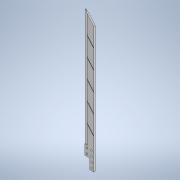
# Autodesk Inventor part: blade D 3.25
Saved by Autodesk Inventor 2021 (Build 250183000, 183)
## iProperties
Created: 2021-04-14
Part Number: blade D 3.25
Material: Generic
Document SubType Name: Modeling
Designer: newic
Density: 1 g/cm^3
Appearance: Default
Author: newic
Autodesk Inventor part; units mm, degrees
ref_plane "YZ Plane" through (0, 0, 0) normal (1, 0, 0) x (0, 1, 0)
ref_plane "XZ Plane" through (0, 0, 0) normal (0, 1, 0) x (-1, 0, 0)
ref_plane "XY Plane" through (0, 0, 0) normal (0, 0, 1) x (1, 0, 0)
sketch "Sketch1" plane through (0, 0, 0) normal (0, 0, 1) x (1, 0, 0)
  line L0 (0, 0) -> (82.55, 0)
  line L1 (82.55, 0) -> (82.55, 968.4207)
  line L2 (82.55, 968.4207) -> (82.55, 804.8513)
  line L3 (82.55, 804.8513) -> (82.55, 621.9713)
  line L4 (82.55, 621.9713) -> (82.55, 439.0913)
  line L5 (82.55, 439.0913) -> (82.55, 256.2113)
  line L6 (82.55, 256.2113) -> (82.55, 73.3313)
  line L7 (0, 1066.8) -> (0, 0)
  line L8 (0, 1066.8) -> (82.55, 968.4207)
  line L9 (-23.6845, 1095.0261) -> (784.1067, 132.338)
  line L10 (-109.2976, 1023.1881) -> (698.4936, 60.5001)
  line L11 (-194.9107, 951.3502) -> (612.8804, -11.3378)
  line L12 (-280.5239, 879.5122) -> (527.2673, -83.1758)
  line L13 (-366.137, 807.6743) -> (441.6542, -155.0137)
  line L14 (-451.7501, 735.8363) -> (356.041, -226.8517)
  dimension "d26" = 1066.8
  dimension "d27" = 82.55
  dimension "d28" = 40
  dimension "d34" = 111.76
  dimension "d35" = 111.76
  dimension "d36" = 111.76
  dimension "d37" = 111.76
  dimension "d38" = 111.76
  constraints: 30 end point, 6 parallel, 6 point on line, 1 horizontal, 1 perpendicular
  measures "d26" distance of L7.start L0.start
  measures "d27" distance of L0.start L0.end
  measures "d28" angle of L8 L1
  measures "d34" distance between parallel lines of L9 L10
  measures "d35" distance between parallel lines of L10 L11
  measures "d36" distance between parallel lines of L11 L12
  measures "d37" distance between parallel lines of L12 L13
  measures "d38" distance between parallel lines of L13 L14
extrude "Extrusion1" add sketch "Sketch1" along normal blind 12.7
sketch "Sketch2" plane through (0, 0, 12.7) normal (0, 0, 1) x (1, 0, 0)
  line L0 (0, 0) -> (82.55, 0)
  line L1 (82.55, 0) -> (82.55, 968.4207)
  line L2 (82.55, 968.4207) -> (82.55, 804.8513)
  line L3 (82.55, 804.8513) -> (82.55, 621.9713)
  line L4 (82.55, 621.9713) -> (82.55, 439.0913)
  line L5 (82.55, 439.0913) -> (82.55, 256.2113)
  line L6 (82.55, 256.2113) -> (82.55, 73.3313)
  line L7 (0, 1066.8) -> (0, 0)
  line L8 (0, 1066.8) -> (82.55, 968.4207)
  line L9 (-23.6845, 1095.0261) -> (784.1067, 132.338)
  line L10 (-109.2976, 1023.1881) -> (698.4936, 60.5001)
  line L11 (-194.9107, 951.3502) -> (612.8804, -11.3378)
  line L12 (-280.5239, 879.5122) -> (527.2673, -83.1758)
  line L13 (-366.137, 807.6743) -> (441.6542, -155.0137)
  line L14 (-451.7501, 735.8363) -> (356.041, -226.8517)
  line L15 (-453.2094, 734.6118) -> (354.5817, -228.0762)
  line L16 (-450.2908, 737.0609) -> (357.5004, -225.6272)
  line L17 (-367.5963, 806.4498) -> (440.1949, -156.2382)
  line L18 (-364.6777, 808.8988) -> (443.1135, -153.7892)
  line L19 (-281.9832, 878.2877) -> (525.808, -84.4003)
  line L20 (-279.0645, 880.7367) -> (528.7266, -81.9513)
  line L21 (-196.37, 950.1257) -> (611.4211, -12.5624)
  line L22 (-193.4514, 952.5747) -> (614.3397, -10.1133)
  line L23 (-110.7569, 1021.9636) -> (697.0342, 59.2756)
  line L24 (-107.8383, 1024.4126) -> (699.9529, 61.7246)
  point P0 (0, 889.9687)
  point P1 (82.55, 791.5894)
  point P2 (82.55, 797.5167)
  point P3 (0, 895.896)
  point P4 (0, 716.101)
  point P5 (82.55, 617.7217)
  point P6 (82.55, 623.649)
  point P7 (0, 722.0283)
  point P8 (0, 542.2333)
  point P9 (82.55, 443.854)
  point P10 (82.55, 449.7813)
  point P11 (0, 548.1606)
  point P12 (0, 368.3656)
  point P13 (82.55, 269.9863)
  point P14 (82.55, 275.9136)
  point P15 (0, 374.2929)
  point P16 (0, 194.4979)
  point P17 (82.55, 96.1186)
  point P18 (82.55, 102.0459)
  point P19 (0, 200.4252)
  dimension "d41" = 1066.8
  dimension "d42" = 82.55
  dimension "d43" = 40
  dimension "d44" = 111.76
  dimension "d45" = 111.76
  dimension "d46" = 111.76
  dimension "d47" = 111.76
  dimension "d48" = 111.76
  dimension "d49" = 1.905
  dimension "d50" = 1.905
  dimension "d51" = 1.905
  dimension "d52" = 1.905
  dimension "d53" = 1.905
  dimension "d54" = 1.905
  dimension "d55" = 1.905
  dimension "d56" = 1.905
  dimension "d57" = 1.905
  dimension "d58" = 1.905
  constraints: 50 end point, 16 parallel, 6 point on line, 1 horizontal, 1 perpendicular
  measures "d41" distance of L7.start L0.start
  measures "d42" distance of L0.start L0.end
  measures "d43" angle of L8 L1
  measures "d44" distance between parallel lines of L9 L10
  measures "d45" distance between parallel lines of L10 L11
  measures "d46" distance between parallel lines of L11 L12
  measures "d47" distance between parallel lines of L12 L13
  measures "d48" distance between parallel lines of L13 L14
  measures "d49" distance between parallel lines of L14 L15
  measures "d50" distance between parallel lines of L14 L16
  measures "d51" distance between parallel lines of L13 L17
  measures "d52" distance between parallel lines of L13 L18
  measures "d53" distance between parallel lines of L12 L19
  measures "d54" distance between parallel lines of L12 L20
  measures "d55" distance between parallel lines of L11 L21
  measures "d56" distance between parallel lines of L11 L22
  measures "d57" distance between parallel lines of L10 L23
  measures "d58" distance between parallel lines of L10 L24
extrude "Extrusion2" cut sketch "Sketch2" against normal blind 12.7 contours L7 L14 L1 L15 | L7 L16 L1 L14 | L7 L13 L1 L17 | L7 L18 L1 L13 | L7 L12 L1 L19 | L7 L20 L1 L12 | L7 L11 L1 L21 | L7 L22 L1 L11 | L7 L10 L1 L23 | L7 L24 L1 L10
sketch "Sketch3" plane through (0, 0, 12.7) normal (0, 0, 1) x (1, 0, 0)
  line L0 (0, 0) -> (82.55, 0)
  line L1 (82.55, 0) -> (82.55, 968.4207)
  line L2 (82.55, 968.4207) -> (82.55, 804.8513)
  line L3 (82.55, 804.8513) -> (82.55, 621.9713)
  line L4 (82.55, 621.9713) -> (82.55, 439.0913)
  line L5 (82.55, 439.0913) -> (82.55, 256.2113)
  line L6 (82.55, 256.2113) -> (82.55, 73.3313)
  line L7 (0, 1066.8) -> (0, 0)
  line L8 (0, 1066.8) -> (82.55, 968.4207)
  line L9 (-23.6845, 1095.0261) -> (784.1067, 132.338)
  line L10 (-109.2976, 1023.1881) -> (698.4936, 60.5001)
  line L11 (-194.9107, 951.3502) -> (612.8804, -11.3378)
  line L12 (-280.5239, 879.5122) -> (527.2673, -83.1758)
  line L13 (-366.137, 807.6743) -> (441.6542, -155.0137)
  line L14 (-451.7501, 735.8363) -> (356.041, -226.8517)
  line L15 (-453.2094, 734.6118) -> (354.5817, -228.0762)
  line L16 (-450.2908, 737.0609) -> (357.5004, -225.6272)
  line L17 (-367.5963, 806.4498) -> (440.1949, -156.2382)
  line L18 (-364.6777, 808.8988) -> (443.1135, -153.7892)
  line L19 (-281.9832, 878.2877) -> (525.808, -84.4003)
  line L20 (-279.0645, 880.7367) -> (528.7266, -81.9513)
  line L21 (-196.37, 950.1257) -> (611.4211, -12.5624)
  line L22 (-193.4514, 952.5747) -> (614.3397, -10.1133)
  line L23 (-110.7569, 1021.9636) -> (697.0342, 59.2756)
  line L24 (-107.8383, 1024.4126) -> (699.9529, 61.7246)
  point P0 (0, 889.9687)
  point P1 (82.55, 791.5894)
  point P2 (82.55, 797.5167)
  point P3 (0, 895.896)
  point P4 (0, 716.101)
  point P5 (82.55, 617.7217)
  point P6 (82.55, 623.649)
  point P7 (0, 722.0283)
  point P8 (0, 542.2333)
  point P9 (82.55, 443.854)
  point P10 (82.55, 449.7813)
  point P11 (0, 548.1606)
  point P12 (0, 368.3656)
  point P13 (82.55, 269.9863)
  point P14 (82.55, 275.9136)
  point P15 (0, 374.2929)
  point P16 (0, 194.4979)
  point P17 (82.55, 96.1186)
  point P18 (82.55, 102.0459)
  point P19 (0, 200.4252)
  point P20 (0, 889.9687)
  point P21 (82.55, 791.5894)
  point P22 (82.55, 797.5167)
  point P23 (0, 895.896)
  point P24 (0, 716.101)
  point P25 (82.55, 617.7217)
  point P26 (82.55, 623.649)
  point P27 (0, 722.0283)
  point P28 (0, 542.2333)
  point P29 (82.55, 443.854)
  point P30 (82.55, 449.7813)
  point P31 (0, 548.1606)
  point P32 (0, 368.3656)
  point P33 (82.55, 269.9863)
  point P34 (82.55, 275.9136)
  point P35 (0, 374.2929)
  point P36 (0, 194.4979)
  point P37 (82.55, 96.1186)
  point P38 (82.55, 102.0459)
  point P39 (0, 200.4252)
  dimension "d114" = 15.875
  dimension "d61" = 1066.8
  dimension "d62" = 82.55
  dimension "d63" = 40
  dimension "d64" = 111.76
  dimension "d65" = 111.76
  dimension "d66" = 111.76
  dimension "d67" = 111.76
  dimension "d68" = 111.76
  dimension "d69" = 1.905
  dimension "d70" = 1.905
  dimension "d71" = 1.905
  dimension "d72" = 1.905
  dimension "d73" = 1.905
  dimension "d74" = 1.905
  dimension "d75" = 1.905
  dimension "d76" = 1.905
  dimension "d77" = 1.905
  dimension "d78" = 1.905
  constraints: 50 end point, 16 parallel, 6 point on line, 1 horizontal, 1 perpendicular
  measures "d61" distance of L7.start L0.start
  measures "d62" distance of L0.start L0.end
  measures "d63" angle of L8 L1
  measures "d64" distance between parallel lines of L9 L10
  measures "d65" distance between parallel lines of L10 L11
  measures "d66" distance between parallel lines of L11 L12
  measures "d67" distance between parallel lines of L12 L13
  measures "d68" distance between parallel lines of L13 L14
  measures "d69" distance between parallel lines of L14 L15
  measures "d70" distance between parallel lines of L14 L16
  measures "d71" distance between parallel lines of L13 L17
  measures "d72" distance between parallel lines of L13 L18
  measures "d73" distance between parallel lines of L12 L19
  measures "d74" distance between parallel lines of L12 L20
  measures "d75" distance between parallel lines of L11 L21
  measures "d76" distance between parallel lines of L11 L22
  measures "d77" distance between parallel lines of L10 L23
  measures "d78" distance between parallel lines of L10 L24
extrude "Extrusion3" add sketch "Sketch3" against normal blind 11.43 contours L7 L14 L1 L15 | L7 L16 L1 L14 | L7 L13 L1 L17 | L7 L18 L1 L13 | L7 L12 L1 L19 | L7 L20 L1 L12 | L7 L11 L1 L21 | L7 L22 L1 L11 | L7 L10 L1 L23 | L7 L24 L1 L10
sketch "Sketch4" plane through (0, 0, 12.7) normal (0, 0, 1) x (1, 0, 0)
  line L0 (0, 0) -> (82.55, 0)
  line L1 (82.55, 0) -> (82.55, 968.4207)
  line L2 (82.55, 968.4207) -> (82.55, 804.8513)
  line L3 (82.55, 804.8513) -> (82.55, 621.9713)
  line L4 (82.55, 621.9713) -> (82.55, 439.0913)
  line L5 (82.55, 439.0913) -> (82.55, 256.2113)
  line L6 (82.55, 256.2113) -> (82.55, 73.3313)
  line L7 (0, 1066.8) -> (0, 0)
  line L8 (0, 1066.8) -> (82.55, 968.4207)
  line L9 (-23.6845, 1095.0261) -> (784.1067, 132.338)
  line L10 (-109.2976, 1023.1881) -> (698.4936, 60.5001)
  line L11 (-194.9107, 951.3502) -> (612.8804, -11.3378)
  line L12 (-280.5239, 879.5122) -> (527.2673, -83.1758)
  line L13 (-366.137, 807.6743) -> (441.6542, -155.0137)
  line L14 (-451.7501, 735.8363) -> (356.041, -226.8517)
  line L15 (-453.2094, 734.6118) -> (354.5817, -228.0762)
  line L16 (-450.2908, 737.0609) -> (357.5004, -225.6272)
  line L17 (-367.5963, 806.4498) -> (440.1949, -156.2382)
  line L18 (-364.6777, 808.8988) -> (443.1135, -153.7892)
  line L19 (-281.9832, 878.2877) -> (525.808, -84.4003)
  line L20 (-279.0645, 880.7367) -> (528.7266, -81.9513)
  line L21 (-196.37, 950.1257) -> (611.4211, -12.5624)
  line L22 (-193.4514, 952.5747) -> (614.3397, -10.1133)
  line L23 (-110.7569, 1021.9636) -> (697.0342, 59.2756)
  line L24 (-107.8383, 1024.4126) -> (699.9529, 61.7246)
  point P0 (0, 889.9687)
  point P1 (82.55, 791.5894)
  point P2 (82.55, 797.5167)
  point P3 (0, 895.896)
  point P4 (0, 716.101)
  point P5 (82.55, 617.7217)
  point P6 (82.55, 623.649)
  point P7 (0, 722.0283)
  point P8 (0, 542.2333)
  point P9 (82.55, 443.854)
  point P10 (82.55, 449.7813)
  point P11 (0, 548.1606)
  point P12 (0, 368.3656)
  point P13 (82.55, 269.9863)
  point P14 (82.55, 275.9136)
  point P15 (0, 374.2929)
  point P16 (0, 194.4979)
  point P17 (82.55, 96.1186)
  point P18 (82.55, 102.0459)
  point P19 (0, 200.4252)
  point P20 (0, 889.9687)
  point P21 (82.55, 791.5894)
  point P22 (82.55, 797.5167)
  point P23 (0, 895.896)
  point P24 (0, 716.101)
  point P25 (82.55, 617.7217)
  point P26 (82.55, 623.649)
  point P27 (0, 722.0283)
  point P28 (0, 542.2333)
  point P29 (82.55, 443.854)
  point P30 (82.55, 449.7813)
  point P31 (0, 548.1606)
  point P32 (0, 368.3656)
  point P33 (82.55, 269.9863)
  point P34 (82.55, 275.9136)
  point P35 (0, 374.2929)
  point P36 (0, 194.4979)
  point P37 (82.55, 96.1186)
  point P38 (82.55, 102.0459)
  point P39 (0, 200.4252)
  dimension "d81" = 1066.8
  dimension "d82" = 82.55
  dimension "d83" = 40
  dimension "d84" = 111.76
  dimension "d85" = 111.76
  dimension "d86" = 111.76
  dimension "d87" = 111.76
  dimension "d88" = 111.76
  dimension "d89" = 1.905
  dimension "d90" = 1.905
  dimension "d91" = 1.905
  dimension "d92" = 1.905
  dimension "d93" = 1.905
  dimension "d94" = 1.905
  dimension "d95" = 1.905
  dimension "d96" = 1.905
  dimension "d97" = 1.905
  dimension "d98" = 1.905
  constraints: 50 end point, 16 parallel, 6 point on line, 1 horizontal, 1 perpendicular
  measures "d81" distance of L7.start L0.start
  measures "d82" distance of L0.start L0.end
  measures "d83" angle of L8 L1
  measures "d84" distance between parallel lines of L9 L10
  measures "d85" distance between parallel lines of L10 L11
  measures "d86" distance between parallel lines of L11 L12
  measures "d87" distance between parallel lines of L12 L13
  measures "d88" distance between parallel lines of L13 L14
  measures "d89" distance between parallel lines of L14 L15
  measures "d90" distance between parallel lines of L14 L16
  measures "d91" distance between parallel lines of L13 L17
  measures "d92" distance between parallel lines of L13 L18
  measures "d93" distance between parallel lines of L12 L19
  measures "d94" distance between parallel lines of L12 L20
  measures "d95" distance between parallel lines of L11 L21
  measures "d96" distance between parallel lines of L11 L22
  measures "d97" distance between parallel lines of L10 L23
  measures "d98" distance between parallel lines of L10 L24
extrude "Extrusion4" cut sketch "Sketch4" against normal blind 1.27 contours L7 L14 L1 L15 | L7 L16 L1 L14 | L7 L13 L1 L17 | L7 L18 L1 L13 | L7 L12 L1 L19 | L7 L20 L1 L12 | L7 L11 L1 L21 | L7 L22 L1 L11 | L7 L10 L1 L23 | L7 L24 L1 L10
sketch "Sketch5" plane through (0, 0, 0) normal (0, -1, 0) x (1, 0, 0)
  line L0 (0, 12.7) -> (82.55, 12.7) projected
  line L1 (0, 12.7) -> (25.4, 12.7)
  line L2 (25.4, 12.7) -> (0, 6.35)
  line L3 (0, 0) -> (0, 12.7) projected
  line L4 (0, 6.35) -> (25.4, 0)
  line L5 (0, 0) -> (82.55, 0) projected
  dimension "d101" = 25.4
  constraints: 6 end point, 2 point on line, 1 midpoint
  measures "d101" distance of L0.start L1.end
extrude "Extrusion5" cut sketch "Sketch5" against normal through all
sketch "Sketch6" plane through (0, 0, 12.7) normal (0, 0, 1) x (1, 0, 0)
  line L0 (25.4, 164.2273) -> (25.4, 0) projected
  line L1 (25.4, 0) -> (82.55, 0) projected
  line L2 (82.55, 0) -> (82.55, 96.1186) projected
  line L3 (82.55, 96.1186) -> (25.4, 164.2273) projected
  line L4 (0, 0) -> (82.55, 0)
  line L5 (82.55, 0) -> (82.55, -91.44)
  line L6 (82.55, -91.44) -> (0, -91.44)
  line L7 (0, -91.44) -> (0, 0)
  line L8 (0, -91.44) -> (45.72, -91.44)
  line L9 (45.72, -91.44) -> (45.72, -182.88)
  line L10 (82.55, -91.44) -> (45.72, -91.44)
  line L11 (45.72, -91.44) -> (45.72, -182.88)
  line L12 (45.72, -182.88) -> (82.55, -182.88)
  line L13 (82.55, -182.88) -> (82.55, -91.44)
  line L14 (0, -45.72) -> (82.55, -45.72)
  line L15 (25.4, 0) -> (82.55, 0) projected
  line L16 (41.275, 0) -> (41.275, -91.44)
  line L17 (45.72, -137.16) -> (82.55, -137.16)
  line L18 (0, -91.44) -> (0, -45.72)
  line L19 (0, -91.44) -> (41.275, -91.44)
  line L20 (41.275, -91.44) -> (82.55, -91.44)
  line L21 (82.55, -91.44) -> (82.55, -45.72)
  line L22 (82.55, -45.72) -> (82.55, 0)
  line L23 (82.55, 0) -> (41.275, 0)
  line L24 (25.4, 0) -> (0, 0) projected
  line L25 (41.275, 0) -> (0, 0)
  line L26 (82.55, -91.44) -> (82.55, -137.16)
  line L27 (45.72, -137.16) -> (45.72, -182.88)
  circle A0 centre (20.6375, -22.86) radius 7.9375
  circle A1 centre (61.9125, -22.86) radius 7.9375
  circle A2 centre (61.9125, -68.58) radius 7.9375
  circle A3 centre (20.6375, -68.58) radius 7.9375
  circle A4 centre (64.135, -114.3) radius 7.9375
  circle A5 centre (64.135, -160.02) radius 7.9375
  dimension "d104" = 91.44
  dimension "d106" = 91.44
  dimension "d107" = 45.72
  dimension "d108" = 91.44
  dimension "d109" = 36.83
  dimension "d110" = 15.875
  dimension "d111" = 15.875
  dimension "d112" = 15.875
  dimension "d113" = 15.875
  dimension "d114" = 15.875
  dimension "d115" = 15.875
  constraints: 44 end point, 6 centre point, 6 coincident, 6 perpendicular, 5 collinear, 5 parallel, 4 midpoint, 3 horizontal, 2 point on line
  measures "d104" distance of L4.end L5.end
  measures "d106" distance of L6.end L4.start
  measures "d107" distance of L8.end L6.end
  measures "d108" distance of L8.end L9.end
  measures "d109" distance of L9.end L12.end
  measures "d110" diameter of A0
  measures "d111" diameter of A1
  measures "d112" diameter of A2
  measures "d113" diameter of A3
  measures "d114" diameter of A4
  measures "d115" diameter of A5
extrude "Extrusion6" add sketch "Sketch6" against normal blind 12.7 contours L1 L16 L14 L7 L4 | L1 L5 L14 L16 | L16 L6 L7 L14 | L14 L5 L6 L16 | L13 L17 L9 L6 | L13 L12 L9 L17
body "Solid1"
